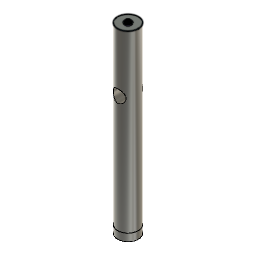
Leg_Assembly v1 (Autodesk Fusion 360 archive; units mm, degrees)
design "Leg_Link_2"
Autodesk Fusion 360 part; units mm, degrees
sketch "Sketch1" plane through (0, 0, 0) normal (0, 0, 1) x (1, 0, 0)
  circle A0 centre (0, 0) radius 4.5
  circle A1 centre (0, 0) radius 1.5
  dimension "d1" = 9
  dimension "d2" = 3
  constraint coincident A0.centre A1.centre
  constraint concentric A0 A1
  measures "d1" diameter of A0
  measures "d2" diameter of A1
extrude "Extrude1" add sketch "Sketch1" against normal blind 76.2 contours A0 | A1 makes body 1
extrude "Extrude2" cut sketch "Sketch1" against normal blind 10 contours A1 bodies 1
sketch "Sketch2" plane through (0, 0, -76.2) normal (0, 0, -1) x (1, 0, 0)
  circle A0 centre (0, 0) radius 4.5
  circle A1 centre (0, 0) radius 1.5
extrude "Extrude3" cut sketch "Sketch2" along normal blind -10 and the other way blind -5 contours A1 bodies 1
ref_plane "WorkPlane1" through (0, 0, 0) normal (0, 1, 0) x (0, 0, 1)
sketch "Sketch3" plane through (0, 0, 0) normal (0, 1, 0) x (1, 0, 0)
  line L0 (4.5, 76.2) -> (-4.5, 76.2)
  line L1 (-4.5, 0) -> (4.5, 0)
  circle A0 centre (0, 25.4) radius 2.75
  line L2 (-4.5, 0) -> (4.5, 0)
  circle A1 centre (0, 81) radius 4.7625
  line L3 (-4.5, 79.4407) -> (-4.5, 76.2)
  arc A2 (-4.5, 79.4407) -> (0, 76.2) centre (0.0531, 81.0184) ccw
  dimension "d10" = 5.5
  dimension "d13" = 25.4
  dimension "d14" = 9.525
  constraint coincident A1 L3.start
  constraint coincident L0.end L3.end
  constraint perpendicular L0 L3
  constraint tangent A1 A2
  constraint midpoint L0 A2.end
  measures "d10" diameter of A0
  measures "d13" distance of A0.centre L2
  measures "d14" diameter of A1
extrude "Extrude4" cut sketch "Sketch3" along normal through all and the other way through all contours A0 bodies 1
revolve "Revolve1" add sketch "Sketch3" angle 360 about axis through (0, 0, 1.75) along (0, 0, 1) separate body contours L0 L3 A2 makes body 2
extrude "Extrude5" cut sketch "Sketch2" along normal blind 5 contours A1 bodies 2
equation "d3 = -25.4 * 3 mm"
equation "d14 = ( ( 3 / 8 ) * 25.4 ) * 1 mm"

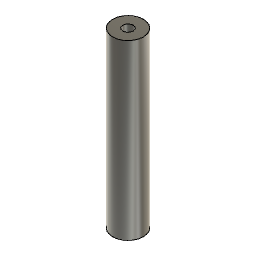
design "Leg_Link_1"
Autodesk Fusion 360 part; units mm, degrees
sketch "Sketch1" plane through (0, 0, 0) normal (0, 0, 1) x (1, 0, 0)
  circle A0 centre (0, 0) radius 4.5
  circle A1 centre (0, 0) radius 1.5
  dimension "d1" = 9
  dimension "d2" = 3
  constraint coincident A0.centre A1.centre
  constraint concentric A0 A1
  measures "d1" diameter of A0
  measures "d2" diameter of A1
extrude "Extrude1" add sketch "Sketch1" against normal blind 50.8 contours A0 | A1
extrude "Extrude2" cut sketch "Sketch1" against normal blind 10 contours A1
sketch "Sketch2" plane through (0, 0, -50.8) normal (0, 0, -1) x (1, 0, 0)
  circle A0 centre (0, 0) radius 4.5
  circle A1 centre (0, 0) radius 1.5
extrude "Extrude3" cut sketch "Sketch2" against normal blind 10 contours A1
equation "d3 = -25.4 * 2 mm"

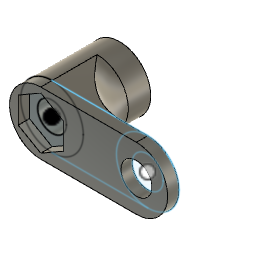
design "End_Cap_Link_New"
Autodesk Fusion 360 part; units mm, degrees
sketch "Sketch1" plane through (0, 0, 0) normal (0, 1, 0) x (1, 0, 0)
  circle A0 centre (0, 0) radius 2.55
  circle A1 centre (17, 0) radius 2.75
  circle A2 centre (0, 0) radius 5.55
  circle A3 centre (17, 0) radius 5.55
  line L0 (0.0003, -5.55) -> (17, -5.55)
  line L1 (0.0003, 5.55) -> (17, 5.55)
  dimension "d1" = 5.1
  dimension "d2" = 5.5
  dimension "d3" = 17
  dimension "d4" = 3
  dimension "d5" = 2.8
  constraint coincident A0.centre A2.centre
  constraint coincident A2 L0.start
  constraint coincident A3 L0.end
  constraint tangent A3 L0
  constraint coincident A2 L1.start
  constraint coincident A3 L1.end
  constraint tangent A3 L1
  measures "d1" diameter of A0
  measures "d2" diameter of A1
  measures "d3" distance of A0.centre A1.centre
extrude "Extrude1" add sketch "Sketch1" along normal blind 12 contours A2
extrude "Extrude2" add sketch "Sketch1" against normal blind 2
fillet "Fillet1" radius 8 1 edges at (5.55, 0, 0)
sketch "Sketch2" plane through (0, -2, 0) normal (0, -1, 0) x (1, 0, 0)
  circle A0 centre (0, 0) radius 2.55
  circle A1 centre (17, 0) radius 2.75
  line L0 (0.0003, -5.55) -> (17, -5.55)
  arc A2 (17, -5.55) -> (17, 5.55) centre (17, 0) ccw
  line L1 (17, 5.55) -> (0.0003, 5.55)
  arc A3 (0.0003, 5.55) -> (0.0003, -5.55) centre (0, 0) ccw
  line L2 (4, 2.3094) -> (0, 4.6188)
  line L3 (0, 4.6188) -> (-4, 2.3094)
  line L4 (-4, 2.3094) -> (-4, -2.3094)
  line L5 (-4, -2.3094) -> (0, -4.6188)
  line L6 (0, -4.6188) -> (4, -2.3094)
  line L7 (4, -2.3094) -> (4, 2.3094)
  line L8 (-4.01, -2.3152) -> (0, -4.6303)
  line L9 (0, -4.6303) -> (4.01, -2.3152)
  line L10 (4.01, -2.3152) -> (4.01, 2.3152)
  line L11 (4.01, 2.3152) -> (0, 4.6303)
  line L12 (0, 4.6303) -> (-4.01, 2.3152)
  line L13 (-4.01, 2.3152) -> (-4.01, -2.3152)
  dimension "d12" = 0.01
  constraint coincident A0.centre A3.centre
extrude "Extrude3" cut sketch "Sketch2" against normal blind 2 contours L2 L3 L4 L5 L6 L7 | L8 L9 L10 L11 L12 L13
equation "d1 = 5 mm + 0.1 mm"
equation "d2 = 5 mm + 0.5 mm"

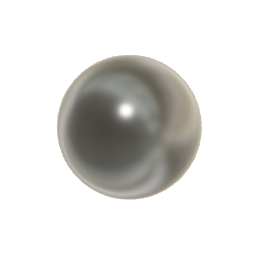
design "Foot_Contact"
Autodesk Fusion 360 part; units mm, degrees
sketch "Sketch1" plane through (0, 0, 0) normal (0, 1, 0) x (1, 0, 0)
  circle A0 centre (0, 0) radius 1.5
  dimension "d1" = 3
  constraint coincident A0.centre origin
  measures "d1" diameter of A0
sphere "SpherePrimitive1" add diameter 9.525 placed x (1, 0, 0) y (0, 0, -1) z (0, 1, 0) at (0, 0, 0)
extrude "Extrude1" cut sketch "Sketch1" along normal blind 5
equation "d2 = ( 3 / 8 ) * 25.4 mm"

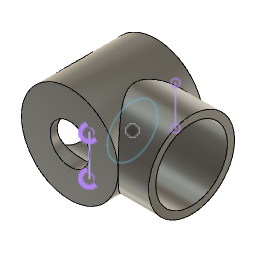
design "End_Cap_Through"
Autodesk Fusion 360 part; units mm, degrees
sketch "Sketch1" plane through (0, 0, 0) normal (0, 1, 0) x (1, 0, 0)
  circle A0 centre (0, 0) radius 2.75
  circle A1 centre (0, 0) radius 6.75
  dimension "d1" = 5.5
  dimension "d2" = 4
  constraint coincident A0.centre A1.centre
  measures "d1" diameter of A0
extrude "Extrude1" add sketch "Sketch1" along normal blind 12
ref_plane "WorkPlane1" through (3, 0, 0) normal (1, 0, 0) x (0, 1, 0)
sketch "Sketch2" plane through (3, 0, 0) normal (1, 0, 0) x (0, 1, 0)
  line L0 (12, -6.75) -> (12, 6.75)
  line L1 (0, -6.75) -> (0, 6.75)
  circle A0 centre (6, 0) radius 4.6
  circle A1 centre (6, 0) radius 6
  dimension "d6" = 9.2
  dimension "d7" = 6
  dimension "d8" = 12
  dimension "d9" = 1.4
  measures "d6" diameter of A0
  measures "d7" distance of L1 A0.centre
  measures "d8" distance of L0.end L1.end
extrude "Extrude2" add sketch "Sketch2" along normal blind 8
ref_plane "WorkPlane2" through (2.75, 6.403, 0) normal (-1, 0, 0) x (0, 0, -1)
sketch "Sketch3" plane through (2.75, 6.403, 0) normal (-1, 0, 0) x (0, -1, 0)
  line L0 (-5.597, -2.75) -> (-5.597, 2.75)
  line L1 (6.403, -2.75) -> (6.403, 2.75)
  line L2 (6.403, -2.75) -> (6.403, 2.75)
  line L3 (-5.597, -2.75) -> (-5.597, 2.75)
  circle A0 centre (0.403, 0) radius 3.5
  point P0 (0.403, 0)
  dimension "d13" = 6
  dimension "d14" = 12
  dimension "d20" = 7
  constraint coincident P0 A0.centre
  measures "d13" distance of P0 L2
  measures "d14" distance of L1.start L3
  measures "d20" diameter of A0
hole "Hole1" at (2.75, 6, 0) direction (1, 0, 0) diameter 3 depth 10 tip angle 118 counterbore diameter 7 counterbore depth 2
extrude "Extrude3" cut sketch "Sketch3" along normal blind 14.5
sketch "Sketch4" plane through (11, 0, 0) normal (1, 0, 0) x (0, 1, 0)
  circle A0 centre (6, 0) radius 4.6
  circle A1 centre (6, 0) radius 6
extrude "Extrude4" cut sketch "Sketch4" against normal blind 35.5 contours A0
sketch "Sketch5" plane through (11, 0, 0) normal (1, 0, 0) x (0, 1, 0)
  circle A0 centre (6, 0) radius 4.6
  circle A1 centre (6, 0) radius 6
  circle A2 centre (6, 0) radius 5
  dimension "d25" = 10
  constraint concentric A0 A2
  measures "d25" diameter of A2
extrude "Extrude5" cut sketch "Sketch5" against normal blind 30 contours A2
equation "d1 = 5 mm + 0.5 mm"
equation "d6 = 9 mm + 0.2 mm"
equation "d7 = d8 / 2"
equation "d13 = d14 / 2"

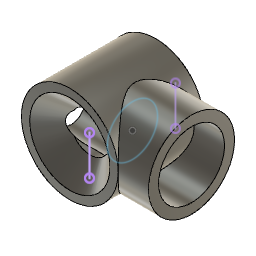
design "End_Cap_Countersink"
Autodesk Fusion 360 part; units mm, degrees
sketch "Sketch1" plane through (0, 0, 0) normal (0, 1, 0) x (1, 0, 0)
  circle A0 centre (0, 0) radius 2.75
  circle A1 centre (0, 0) radius 6.75
  dimension "d1" = 5.5
  dimension "d2" = 4
  constraint coincident A0.centre A1.centre
  measures "d1" diameter of A0
extrude "Extrude1" add sketch "Sketch1" along normal blind 12
ref_plane "WorkPlane1" through (3, 0, 0) normal (1, 0, 0) x (0, 1, 0)
sketch "Sketch2" plane through (3, 0, 0) normal (1, 0, 0) x (0, 1, 0)
  line L0 (12, -6.75) -> (12, 6.75)
  line L1 (0, -6.75) -> (0, 6.75)
  circle A0 centre (6, 0) radius 4.6
  circle A1 centre (6, 0) radius 6
  dimension "d6" = 9.2
  dimension "d7" = 6
  dimension "d8" = 12
  dimension "d9" = 1.4
  measures "d6" diameter of A0
  measures "d7" distance of L1 A0.centre
  measures "d8" distance of L0.end L1.end
extrude "Extrude2" add sketch "Sketch2" along normal blind 8
ref_plane "WorkPlane2" through (2.75, 6.403, 0) normal (-1, 0, 0) x (0, 0, -1)
sketch "Sketch3" plane through (2.75, 6.403, 0) normal (-1, 0, 0) x (0, -1, 0)
  line L0 (-5.597, -2.75) -> (-5.597, 2.75)
  line L1 (6.403, -2.75) -> (6.403, 2.75)
  line L2 (6.403, -2.75) -> (6.403, 2.75)
  line L3 (-5.597, -2.75) -> (-5.597, 2.75)
  circle A0 centre (0.403, 0) radius 3.5
  point P0 (0.403, 0)
  dimension "d13" = 6
  dimension "d14" = 12
  dimension "d20" = 7
  constraint coincident P0 A0.centre
  measures "d13" distance of P0 L2
  measures "d14" distance of L1.start L3
  measures "d20" diameter of A0
hole "Hole1" at (2.75, 6, 0) direction (1, 0, 0) diameter 3 depth 10 tip angle 118 counterbore diameter 7 counterbore depth 2
extrude "Extrude3" cut sketch "Sketch3" along normal blind 14.5
sketch "Sketch4" plane through (0, 0, 0) normal (0, 1, 0) x (1, 0, 0)
hole "Hole2" at (0, 0, 0) direction (0, 1, 0) diameter 5.5 depth 25.5 tip angle 118 countersink diameter 11.2 countersink angle 90
equation "d1 = 5 mm + 0.5 mm"
equation "d6 = 9 mm + 0.2 mm"
equation "d7 = d8 / 2"
equation "d13 = d14 / 2"

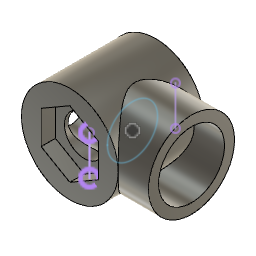
design "End_Cap_1"
Autodesk Fusion 360 part; units mm, degrees
sketch "Sketch1" plane through (0, 0, 0) normal (0, 1, 0) x (1, 0, 0)
  circle A0 centre (0, 0) radius 2.75
  circle A1 centre (0, 0) radius 6.75
  dimension "d1" = 5.5
  dimension "d2" = 4
  constraint coincident A0.centre A1.centre
  measures "d1" diameter of A0
extrude "Extrude1" add sketch "Sketch1" along normal blind 12
ref_plane "WorkPlane1" through (3, 0, 0) normal (1, 0, 0) x (0, 1, 0)
sketch "Sketch2" plane through (3, 0, 0) normal (1, 0, 0) x (0, 1, 0)
  line L0 (12, -6.75) -> (12, 6.75)
  line L1 (0, -6.75) -> (0, 6.75)
  circle A0 centre (6, 0) radius 4.6
  circle A1 centre (6, 0) radius 6
  dimension "d6" = 9.2
  dimension "d7" = 6
  dimension "d8" = 12
  dimension "d9" = 1.4
  measures "d6" diameter of A0
  measures "d7" distance of L1 A0.centre
  measures "d8" distance of L0.end L1.end
extrude "Extrude2" add sketch "Sketch2" along normal blind 8
ref_plane "WorkPlane2" through (2.75, 6.403, 0) normal (-1, 0, 0) x (0, 0, -1)
sketch "Sketch3" plane through (2.75, 6.403, 0) normal (-1, 0, 0) x (0, -1, 0)
  line L0 (-5.597, -2.75) -> (-5.597, 2.75)
  line L1 (6.403, -2.75) -> (6.403, 2.75)
  line L2 (6.403, -2.75) -> (6.403, 2.75)
  line L3 (-5.597, -2.75) -> (-5.597, 2.75)
  circle A0 centre (0.403, 0) radius 3.5
  point P0 (0.403, 0)
  dimension "d13" = 6
  dimension "d14" = 12
  dimension "d20" = 7
  constraint coincident P0 A0.centre
  measures "d13" distance of P0 L2
  measures "d14" distance of L1.start L3
  measures "d20" diameter of A0
hole "Hole1" at (2.75, 6, 0) direction (1, 0, 0) diameter 3 depth 10 tip angle 118 counterbore diameter 7 counterbore depth 2
extrude "Extrude3" cut sketch "Sketch3" along normal blind 14.5
sketch "Sketch4" plane through (0, 0, 0) normal (0, -1, 0) x (1, 0, 0)
  circle A0 centre (0, 0) radius 2.75
  circle A1 centre (0, 0) radius 6.75
  line L0 (4, 2.3094) -> (0, 4.6188)
  line L1 (0, 4.6188) -> (-4, 2.3094)
  line L2 (-4, 2.3094) -> (-4, -2.3094)
  line L3 (-4, -2.3094) -> (0, -4.6188)
  line L4 (0, -4.6188) -> (4, -2.3094)
  line L5 (4, -2.3094) -> (4, 2.3094)
  line L6 (-4.01, -2.3152) -> (0, -4.6303)
  line L7 (0, -4.6303) -> (4.01, -2.3152)
  line L8 (4.01, -2.3152) -> (4.01, 2.3152)
  line L9 (4.01, 2.3152) -> (0, 4.6303)
  line L10 (0, 4.6303) -> (-4.01, 2.3152)
  line L11 (-4.01, 2.3152) -> (-4.01, -2.3152)
  dimension "d23" = 0.01
  constraint coincident A0.centre A1.centre
extrude "Extrude4" cut sketch "Sketch4" against normal blind 2 contours L0 L1 L2 L3 L4 L5 | L6 L7 L8 L9 L10 L11
equation "d1 = 5 mm + 0.5 mm"
equation "d6 = 9 mm + 0.2 mm"
equation "d7 = d8 / 2"
equation "d13 = d14 / 2"
